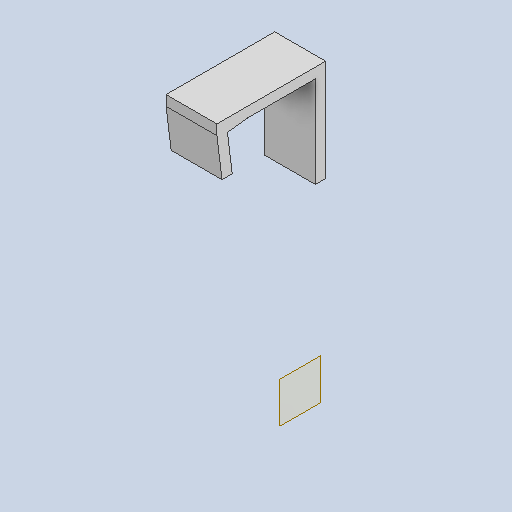
# Autodesk Inventor part: coverHolder_CPY
Saved by Autodesk Inventor 2023 (Build 270158000, 158)
## iProperties
Created: 2023-02-02
Part Number: coverHolder_CPY
Material: Generic
Document SubType Name: Modeling
Designer: shrey
Density: 1 g/cm^3
Appearance: Default
Author: shrey
Autodesk Inventor part; units mm, degrees
ref_plane "XZ Plane" through (0, 0, 0) normal (0, 1, 0) x (-1, 0, 0)
ref_plane "XY Plane" through (0, 0, 0) normal (0, 0, 1) x (1, 0, 0)
ref_plane "Work Plane1" through (78.575, 0, 0) normal (1, 0, 0) x (0, 1, 0)
sketch "Sketch2" plane through (78.575, 0, 0) normal (1, 0, 0) x (0, 1, 0)
  line L0 (-170.29, 0) -> (141.6673, 38.3035) projected
  line L1 (141.6673, 38.3035) -> (140.4486, 48.229) projected
  line L2 (-171.5087, 9.9255) -> (140.4486, 48.229) projected
  line L3 (-170.29, 0) -> (-171.5087, 9.9255) projected
  line L4 (-304.8, 0) -> (304.8, 0) projected
  line L5 (-304.8, 0) -> (-304.8, -25.4) projected
  line L6 (304.8, -25.4) -> (-304.8, -25.4) projected
  line L7 (304.8, 0) -> (304.8, -25.4) projected
  line L8 (141.6673, 0) -> (146.6673, 0)
  line L9 (146.6673, 0) -> (146.6673, 53.4221)
  line L10 (146.6673, 53.4221) -> (141.6673, 53.4221)
  line L11 (141.6673, 53.4221) -> (141.6673, 0)
  line L12 (141.6673, 53.4221) -> (121.6673, 53.4221)
  line L13 (121.6673, 53.4221) -> (121.6673, 38.3035)
  line L14 (121.6673, 38.3035) -> (141.6673, 38.3035)
  line L15 (141.6673, 38.3035) -> (141.6673, 53.4221)
  line L16 (141.6673, 38.3035) -> (140.4486, 48.229)
  line L17 (121.6673, 45.8628) -> (140.4486, 48.229)
  line L18 (146.6673, 0) -> (96.6673, 0)
  line L19 (96.6673, 0) -> (96.6673, 5)
  line L20 (96.6673, 5) -> (146.6673, 5)
  line L21 (146.6673, 5) -> (146.6673, 0)
  line L22 (141.6673, 53.4221) -> (121.6673, 50.9023)
  line L23 (101.6673, 0) -> (141.6673, 0)
  line L24 (141.6673, 0) -> (141.6673, 0.95)
  line L25 (141.6673, 0.95) -> (101.6673, 0.95)
  line L26 (101.6673, 0.95) -> (101.6673, 0)
  point P0 (0, 0)
  point P1 (141.6673, 5)
  point P2 (121.6673, 45.9229)
  dimension "d2" = 5
  dimension "d3" = 20
  dimension "d4" = 50
  dimension "d5" = 5
  dimension "d6" = 5
  dimension "d7" = 40
  dimension "d8" = 5
  dimension "d9" = 0.95
  constraints: 38 end point, 9 parallel, 4 horizontal, 4 perpendicular, 3 point on line, 1 collinear, 1 midpoint, 1 vertical
  measures "d2" distance of L9.end L10.end
  measures "d3" distance between parallel lines of L11 L13
  measures "d4" distance of L19.end L20.end
  measures "d5" distance of L18.end L19.end
  measures "d6" distance between parallel lines of L22 L17
  measures "d7" distance of L25.end L24.end
  measures "d8" distance between parallel lines of L19 L26
  measures "d9" distance of L25.end L23.start
extrude "Extrusion1" add sketch "Sketch2" along normal mid plane 25 contours L1 L2 L13 L22 L11 | L11 L10 L9 L20 | L19 L20 L11 L25 L26 L4 | L20 L9 L4 L11 | L26 L25 L11 L4
extrude "Extrusion2" cut sketch "Sketch2" along normal mid plane 13.2 contours L26 L25 L11 L4
body "Solid1"
